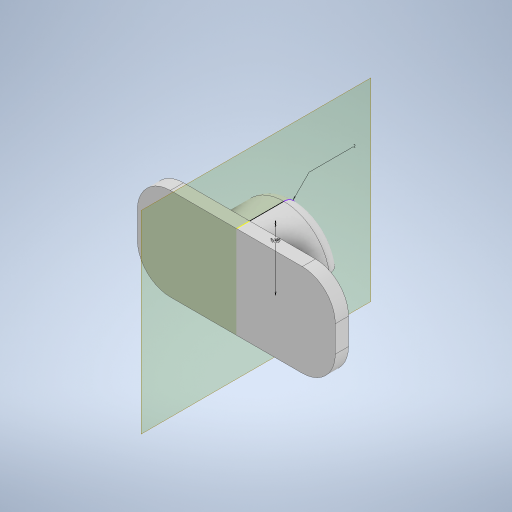
# Autodesk Inventor part: Wheelmount
Saved by Autodesk Inventor 2024 (Build 280153000, 153)
## iProperties
Created: 2024-04-29
Part Number: Wheelmount
Material: Generic
Document SubType Name: Modeling
Designer: Hitesh
Density: 1 g/cm^3
Appearance: Default
Author: Hitesh
Autodesk Inventor part; units mm, degrees
ref_plane "YZ Plane" through (0, 0, 0) normal (1, 0, 0) x (0, 1, 0)
ref_plane "XZ Plane" through (0, 0, 0) normal (0, 1, 0) x (-1, 0, 0)
ref_plane "XY Plane" through (0, 0, 0) normal (0, 0, 1) x (1, 0, 0)
sketch "Sketch1" plane through (0, 0, 0) normal (0, 0, 1) x (1, 0, 0)
  line L0 (5, 0) -> (25, 0)
  line L1 (30, -5) -> (30, -9)
  line L2 (25, -14) -> (5, -14)
  line L3 (0, -9) -> (0, -5)
  arc A0 (0, -9) -> (5, -14) centre (5, -9) ccw
  arc A1 (5, 0) -> (0, -5) centre (5, -5) ccw
  arc A2 (30, -5) -> (25, 0) centre (25, -5) ccw
  arc A3 (25, -14) -> (30, -9) centre (25, -9) ccw
  point P0 (0, 0)
  point P1 (30, -14)
  point P2 (30, 0)
  point P3 (0, -14)
  dimension "d0" = 30
  dimension "d1" = 14
  dimension "d2" = 5
  constraints: 8 end point, 8 point on circle, 8 point on line, 8 tangent, 4 centre point, 3 equal radius, 2 parallel, 1 horizontal, 1 perpendicular
  measures "d0" distance of point (30, -14) point (0, -14)
  measures "d1" distance of point (30, 0) point (30, -14)
  measures "d2" radius of A0
extrude "Extrusion1" add sketch "Sketch1" along normal blind 2
ref_plane "Work Plane1" through (15, -9, 0) normal (-1, 0, 0) x (0, 0, 1)
sketch "Sketch2" plane through (15, -9, 0) normal (-1, 0, 0) x (0, 0, 1)
  circle A0 centre (-3.9426, 2) radius 4.775 construction
  line L0 (-3.9426, 2) -> (0, 2) construction
  line L1 (0, 0) -> (0, 4) construction
  line L2 (0, 4) -> (0, 9) construction
  line L3 (0, 9) -> (-5.1622, 9) construction
  line L4 (-7.1622, 7) -> (-7.1622, 5.2744) construction
  line L5 (-7.1622, 5.2744) -> (0, 5.2744) construction
  line L6 (0, 5.2744) -> (0, 9) construction
  arc A1 (0, 5.2744) -> (-7.1622, 5.9874) centre (-3.9426, 2) ccw
  line L7 (-7.1622, 5.9874) -> (-7.1622, 7)
  line L8 (-5.1622, 9) -> (0, 9)
  line L9 (0, 9) -> (2, 9) projected
  line L10 (0, 9) -> (0, 5.2744)
  arc A2 (-5.1622, 9) -> (-7.1622, 7) centre (-5.1622, 7) ccw
  line L11 (-5.1622, 9) -> (0, 9)
  dimension "d5" = 9.55
  dimension "d6" = 5.125
  dimension "d7" = 2
  constraints: 18 end point, 5 point on circle, 3 centre point, 3 point on line, 3 tangent, 2 collinear, 2 parallel, 2 perpendicular, 1 coincident, 1 horizontal, 1 midpoint, 1 vertical
  measures "d5" diameter of A0
  measures "d6" radius of A1
  measures "d7" radius of A2
revolve "Revolution1" add sketch "Sketch2" angle 360 about axis through (15, -7, -3.9426) along (0, 0, 1)
sketch "Sketch3" plane through (15, -9, 0) normal (-1, 0, 0) x (0, 0, 1)
  line L0 (0, 0) -> (0, 4) projected
  line L1 (-7.1622, -1.9874) -> (-7.1622, 5.9874) projected
  line L2 (0, 2) -> (-7.1622, 2)
  line L3 (-7.1622, 2) -> (-7.1622, 2.9338)
  line L4 (-7.1622, 2.9338) -> (0, 2.9338)
  line L5 (0, 2.9338) -> (0, 2)
  line L6 (-7.1622, 2) -> (0, 2)
  line L7 (0, 2) -> (0, 1.066)
  line L8 (0, 1.066) -> (-7.1622, 1.066)
  line L9 (-7.1622, 1.066) -> (-7.1622, 2)
  point P0 (0, 9)
  point P1 (0, 2.9338)
  point P2 (-7.1622, 1.066)
  dimension "d9" = 0.934
  constraints: 16 end point, 4 parallel, 2 horizontal, 2 perpendicular, 2 point on line, 1 midpoint
  measures "d9" distance of L6.end L7.end
extrude "Extrusion2" cut sketch "Sketch3" along normal through all both and the other way through all
sketch "Sketch4" plane through (15, -9, 0) normal (-1, 0, 0) x (0, 0, 1)
  line L0 (0, 4) -> (0, 9) projected
  arc A0 (1.1539, 2) -> (0, 5.2289) centre (-3.9407, 2) ccw
  line L1 (0, 4) -> (0, 0) projected
  line L2 (0, 2) -> (0, 5.2289)
  line L3 (0, 2) -> (1.1539, 2)
  constraints: 4 end point, 2 point on circle, 2 point on line, 1 centre point, 1 horizontal, 1 midpoint
revolve "Revolution2" cut sketch "Sketch4" angle 360 about axis through (15, -7, -3.9426) along (0, 0, 1)
body "Solid1"
